Autodesk Fusion 360 part; units mm, degrees
note: some values were not read from the file. Set by a fixed rule: which sketch regions a step uses.
(part 57 of 59)
  spline S63 degree 5 poles (29.6298, 3.3854) (29.6276, 3.3871) (29.6234, 3.3904) (29.6169, 3.3953) (29.6084, 3.4019) (29.5977, 3.41) (29.587, 3.4182) (29.5763, 3.4263) (29.5657, 3.4343) (29.555, 3.4424) (29.5444, 3.4504) (29.5338, 3.4584) (29.5232, 3.4663) (29.5127, 3.4742) (29.5021, 3.4821) (29.4915, 3.4899) (29.481, 3.4978) (29.4705, 3.5055) (29.46, 3.5133) (29.4495, 3.521) (29.4391, 3.5287) (29.4286, 3.5363) (29.4182, 3.544) (29.4078, 3.5515) (29.3974, 3.5591) (29.387, 3.5666) (29.3766, 3.5741) (29.3663, 3.5816) (29.356, 3.589) (29.3457, 3.5964) (29.3354, 3.6037) (29.3251, 3.6111) (29.3148, 3.6184) (29.3046, 3.6256) (29.2944, 3.6329) (29.2842, 3.64) (29.274, 3.6472) (29.2638, 3.6543) (29.2537, 3.6614) (29.2435, 3.6685) (29.2334, 3.6755) (29.2233, 3.6825) (29.2132, 3.6895) (29.2032, 3.6964) (29.1932, 3.7033) (29.1831, 3.7102) (29.1731, 3.717) (29.1632, 3.7238) (29.1532, 3.7306) (29.1433, 3.7374) (29.1334, 3.7441) (29.1235, 3.7507) (29.1136, 3.7574) (29.1037, 3.764) (29.0939, 3.7705) (29.0841, 3.7771) (29.0743, 3.7836) (29.0646, 3.7901) (29.0548, 3.7965) (29.0451, 3.8029) (29.0354, 3.8093) (29.0257, 3.8156) (29.016, 3.8219) (29.0064, 3.8282) (28.9968, 3.8344) (28.9872, 3.8407) (28.9776, 3.8468) (28.9681, 3.853) (28.9586, 3.8591) (28.9491, 3.8652) (28.9396, 3.8712) (28.9302, 3.8772) (28.9207, 3.8832) (28.9113, 3.8891) (28.902, 3.895) (28.8926, 3.9009) (28.8833, 3.9068) (28.874, 3.9126) (28.8647, 3.9183) (28.8555, 3.9241) (28.8462, 3.9298) (28.837, 3.9355) (28.8279, 3.9411) (28.8187, 3.9467) (28.8096, 3.9523) (28.8005, 3.9578) (28.7914, 3.9633) (28.7824, 3.9688) (28.7734, 3.9743) (28.7644, 3.9797) (28.7554, 3.985) (28.7465, 3.9904) (28.7376, 3.9957) (28.7287, 4.001) (28.7199, 4.0062) (28.711, 4.0114) (28.7022, 4.0166) (28.6935, 4.0217) (28.6847, 4.0268) (28.676, 4.0319) (28.6674, 4.037) (28.6587, 4.042) (28.6501, 4.0469) (28.6415, 4.0519) (28.633, 4.0568) (28.6244, 4.0616) (28.616, 4.0665) (28.6075, 4.0713) (28.5991, 4.0761) (28.5907, 4.0808) (28.5823, 4.0855) (28.574, 4.0902) (28.5657, 4.0948) (28.5574, 4.0994) (28.5491, 4.104) (28.5409, 4.1085) (28.5328, 4.113) (28.5246, 4.1175) (28.5165, 4.1219) (28.5085, 4.1263) (28.5004, 4.1307) (28.4924, 4.135) (28.4845, 4.1393) (28.4765, 4.1435) (28.4686, 4.1478) (28.4608, 4.152) (28.4529, 4.1561) (28.4452, 4.1602) (28.4374, 4.1643) (28.4297, 4.1684) (28.422, 4.1724) (28.4144, 4.1764) (28.4068, 4.1804) (28.3992, 4.1843) (28.3917, 4.1882) (28.3842, 4.192) (28.3767, 4.1958) (28.3693, 4.1996) (28.3619, 4.2034) (28.3546, 4.2071) (28.3473, 4.2108) (28.3401, 4.2144) (28.3329, 4.218) (28.3257, 4.2216) (28.3186, 4.2252) (28.3115, 4.2287) (28.3044, 4.2322) (28.2974, 4.2356) (28.2905, 4.239) (28.2835, 4.2424) (28.2767, 4.2457) (28.2698, 4.249) (28.263, 4.2523) (28.2563, 4.2555) (28.2496, 4.2588) (28.2429, 4.2619) (28.2363, 4.2651) (28.2298, 4.2682) (28.2233, 4.2712) (28.2168, 4.2743) (28.2104, 4.2773) (28.204, 4.2802) (28.1977, 4.2831) (28.1914, 4.286) (28.1851, 4.2889) (28.179, 4.2917) (28.1728, 4.2945) (28.1667, 4.2973) (28.1607, 4.3) (28.1547, 4.3027) (28.1488, 4.3053) (28.1429, 4.308) (28.1371, 4.3105) (28.1313, 4.3131) (28.1256, 4.3156) (28.1199, 4.3181) (28.1143, 4.3205) (28.1087, 4.323) (28.1032, 4.3253) (28.0978, 4.3277) (28.0924, 4.33) (28.087, 4.3323) (28.0818, 4.3345) (28.0765, 4.3367) (28.0714, 4.3389) (28.0663, 4.341) (28.0612, 4.3431) (28.0562, 4.3452) (28.0513, 4.3472) (28.0464, 4.3492) (28.0416, 4.3512) (28.0369, 4.3531) (28.0322, 4.355) (28.0276, 4.3568) (28.023, 4.3587) (28.0185, 4.3605) (28.0141, 4.3622) (28.0097, 4.3639) (28.0054, 4.3656) (28.0012, 4.3673) (27.997, 4.3689) (27.9929, 4.3705) (27.9889, 4.372) (27.9849, 4.3735) (27.9811, 4.375) (27.9772, 4.3764) (27.9735, 4.3778) (27.9698, 4.3792) (27.9662, 4.3806) (27.9627, 4.3819) (27.9593, 4.3831) (27.9559, 4.3844) (27.9526, 4.3856) (27.9494, 4.3867) (27.9462, 4.3879) (27.9432, 4.3889) (27.9402, 4.39) (27.9373, 4.391) (27.9345, 4.392) (27.9318, 4.393) (27.9291, 4.3939) (27.9265, 4.3948) (27.9241, 4.3956) (27.9217, 4.3964) (27.9194, 4.3972) (27.9172, 4.398) (27.915, 4.3987) (27.913, 4.3993) (27.9111, 4.4) (27.9092, 4.4006) (27.9075, 4.4012) (27.9058, 4.4017) (27.9043, 4.4022) (27.9028, 4.4027) (27.9015, 4.4031) (27.9002, 4.4035) (27.8991, 4.4038) (27.898, 4.4042) (27.8971, 4.4044) (27.8963, 4.4047) (27.8956, 4.4049) (27.8951, 4.4051) (27.8948, 4.4052) (27.8946, 4.4052) (27.8945, 4.4052) knots -1 -1 -1 -1 -1 -1 -0.99583333 -0.99166667 -0.9875 -0.98333333 -0.97916667 -0.975 -0.97083333 -0.96666667 -0.9625 -0.95833333 -0.95416667 -0.95 -0.94583333 -0.94166667 -0.9375 -0.93333333 -0.92916667 -0.925 -0.92083333 -0.91666667 -0.9125 -0.90833333 -0.90416667 -0.9 -0.89583333 -0.89166667 -0.8875 -0.88333333 -0.87916667 -0.875 -0.87083333 -0.86666667 -0.8625 -0.85833333 -0.85416667 -0.85 -0.84583333 -0.84166667 -0.8375 -0.83333333 -0.82916667 -0.825 -0.82083333 -0.81666667 -0.8125 -0.80833333 -0.80416667 -0.8 -0.79583333 -0.79166667 -0.7875 -0.78333333 -0.77916667 -0.775 -0.77083333 -0.76666667 -0.7625 -0.75833333 -0.75416667 -0.75 -0.74583333 -0.74166667 -0.7375 -0.73333333 -0.72916667 -0.725 -0.72083333 -0.71666667 -0.7125 -0.70833333 -0.70416667 -0.7 -0.69583333 -0.69166667 -0.6875 -0.68333333 -0.67916667 -0.675 -0.67083333 -0.66666667 -0.6625 -0.65833333 -0.65416667 -0.65 -0.64583333 -0.64166667 -0.6375 -0.63333333 -0.62916667 -0.625 -0.62083333 -0.61666667 -0.6125 -0.60833333 -0.60416667 -0.6 -0.59583333 -0.59166667 -0.5875 -0.58333333 -0.57916667 -0.575 -0.57083333 -0.56666667 -0.5625 -0.55833333 -0.55416667 -0.55 -0.54583333 -0.54166667 -0.5375 -0.53333333 -0.52916667 -0.525 -0.52083333 -0.51666667 -0.5125 -0.50833333 -0.50416667 -0.5 -0.49583333 -0.49166667 -0.4875 -0.48333333 -0.47916667 -0.475 -0.47083333 -0.46666667 -0.4625 -0.45833333 -0.45416667 -0.45 -0.44583333 -0.44166667 -0.4375 -0.43333333 -0.42916667 -0.425 -0.42083333 -0.41666667 -0.4125 -0.40833333 -0.40416667 -0.4 -0.39583333 -0.39166667 -0.3875 -0.38333333 -0.37916667 -0.375 -0.37083333 -0.36666667 -0.3625 -0.35833333 -0.35416667 -0.35 -0.34583333 -0.34166667 -0.3375 -0.33333333 -0.32916667 -0.325 -0.32083333 -0.31666667 -0.3125 -0.30833333 -0.30416667 -0.3 -0.29583333 -0.29166667 -0.2875 -0.28333333 -0.27916667 -0.275 -0.27083333 -0.26666667 -0.2625 -0.25833333 -0.25416667 -0.25 -0.24583333 -0.24166667 -0.2375 -0.23333333 -0.22916667 -0.225 -0.22083333 -0.21666667 -0.2125 -0.20833333 -0.20416667 -0.2 -0.19583333 -0.19166667 -0.1875 -0.18333333 -0.17916667 -0.175 -0.17083333 -0.16666667 -0.1625 -0.15833333 -0.15416667 -0.15 -0.14583333 -0.14166667 -0.1375 -0.13333333 -0.12916667 -0.125 -0.12083333 -0.11666667 -0.1125 -0.10833333 -0.10416667 -0.1 -0.09583333 -0.09166667 -0.0875 -0.08333333 -0.07916667 -0.075 -0.07083333 -0.06666667 -0.0625 -0.05833333 -0.05416667 -0.05 -0.04583333 -0.04166667 -0.0375 -0.03333333 -0.02916667 -0.025 -0.02083333 -0.01666667 -0.0125 -0.00833333 -0.00416667 0 0 0 0 0 0
  line L127 (27.8945, 4.4052) -> (27.8937, 4.4055)
  line L128 (27.8937, 4.4055) -> (27.6109, 4.4875)
  arc A64 (27.6109, 4.4875) -> (27.918, 5.6335) centre (0, 12.5) ccw
  line L129 (27.918, 5.6335) -> (28.2039, 5.5632)
  line L130 (28.2039, 5.5632) -> (28.2047, 5.563)
  spline S64 degree 5 poles (28.2047, 5.563) (28.2048, 5.563) (28.205, 5.563) (28.2053, 5.5629) (28.2058, 5.5628) (28.2065, 5.5626) (28.2074, 5.5624) (28.2083, 5.5622) (28.2094, 5.5619) (28.2106, 5.5617) (28.2118, 5.5614) (28.2132, 5.5611) (28.2147, 5.5608) (28.2163, 5.5604) (28.218, 5.5601) (28.2198, 5.5597) (28.2217, 5.5593) (28.2237, 5.5589) (28.2258, 5.5584) (28.228, 5.558) (28.2303, 5.5575) (28.2327, 5.5571) (28.2351, 5.5566) (28.2377, 5.5561) (28.2404, 5.5555) (28.2431, 5.555) (28.246, 5.5545) (28.2489, 5.5539) (28.2519, 5.5534) (28.255, 5.5528) (28.2582, 5.5522) (28.2615, 5.5516) (28.2649, 5.551) (28.2683, 5.5504) (28.2719, 5.5498) (28.2755, 5.5492) (28.2792, 5.5485) (28.283, 5.5479) (28.2868, 5.5472) (28.2908, 5.5466) (28.2948, 5.5459) (28.2989, 5.5453) (28.3031, 5.5446) (28.3074, 5.5439) (28.3117, 5.5432) (28.3161, 5.5426) (28.3206, 5.5419) (28.3252, 5.5412) (28.3298, 5.5405) (28.3345, 5.5398) (28.3393, 5.5391) (28.3442, 5.5384) (28.3491, 5.5377) (28.3541, 5.537) (28.3592, 5.5363) (28.3643, 5.5356) (28.3695, 5.5349) (28.3748, 5.5342) (28.3802, 5.5335) (28.3856, 5.5328) (28.3911, 5.5321) (28.3966, 5.5314) (28.4023, 5.5307) (28.408, 5.53) (28.4137, 5.5293) (28.4196, 5.5286) (28.4255, 5.5279) (28.4314, 5.5272) (28.4374, 5.5265) (28.4435, 5.5258) (28.4497, 5.5251) (28.4559, 5.5244) (28.4622, 5.5237) (28.4685, 5.5231) (28.4749, 5.5224) (28.4814, 5.5217) (28.4879, 5.5211) (28.4945, 5.5204) (28.5011, 5.5197) (28.5078, 5.5191) (28.5146, 5.5184) (28.5214, 5.5178) (28.5283, 5.5172) (28.5353, 5.5165) (28.5423, 5.5159) (28.5493, 5.5153) (28.5564, 5.5147) (28.5636, 5.5141) (28.5709, 5.5135) (28.5781, 5.5129) (28.5855, 5.5123) (28.5929, 5.5118) (28.6004, 5.5112) (28.6079, 5.5106) (28.6154, 5.5101) (28.6231, 5.5095) (28.6307, 5.509) (28.6385, 5.5085) (28.6463, 5.5079) (28.6541, 5.5074) (28.662, 5.5069) (28.67, 5.5064) (28.678, 5.506) (28.686, 5.5055) (28.6941, 5.505) (28.7023, 5.5046) (28.7105, 5.5041) (28.7187, 5.5037) (28.727, 5.5032) (28.7354, 5.5028) (28.7438, 5.5024) (28.7523, 5.502) (28.7608, 5.5016) (28.7694, 5.5013) (28.778, 5.5009) (28.7866, 5.5005) (28.7953, 5.5002) (28.8041, 5.4999) (28.8129, 5.4995) (28.8218, 5.4992) (28.8307, 5.4989) (28.8396, 5.4986) (28.8486, 5.4984) (28.8577, 5.4981) (28.8668, 5.4979) (28.8759, 5.4976) (28.8851, 5.4974) (28.8943, 5.4972) (28.9036, 5.497) (28.9129, 5.4968) (28.9223, 5.4966) (28.9317, 5.4964) (28.9412, 5.4963) (28.9507, 5.4962) (28.9602, 5.496) (28.9698, 5.4959) (28.9795, 5.4958) (28.9892, 5.4957) (28.9989, 5.4957) (29.0087, 5.4956) (29.0185, 5.4956) (29.0284, 5.4955) (29.0383, 5.4955) (29.0482, 5.4955) (29.0582, 5.4955) (29.0682, 5.4956) (29.0783, 5.4956) (29.0884, 5.4957) (29.0986, 5.4957) (29.1088, 5.4958) (29.119, 5.4959) (29.1293, 5.496) (29.1396, 5.4962) (29.15, 5.4963) (29.1604, 5.4965) (29.1708, 5.4966) (29.1813, 5.4968) (29.1919, 5.497) (29.2024, 5.4972) (29.213, 5.4975) (29.2237, 5.4977) (29.2344, 5.498) (29.2451, 5.4983) (29.2559, 5.4986) (29.2667, 5.4989) (29.2775, 5.4992) (29.2884, 5.4996) (29.2993, 5.4999) (29.3103, 5.5003) (29.3213, 5.5007) (29.3323, 5.5011) (29.3434, 5.5016) (29.3545, 5.502) (29.3657, 5.5025) (29.3768, 5.503) (29.3881, 5.5035) (29.3993, 5.504) (29.4106, 5.5045) (29.422, 5.505) (29.4333, 5.5056) (29.4447, 5.5062) (29.4562, 5.5068) (29.4677, 5.5074) (29.4792, 5.508) (29.4907, 5.5087) (29.5023, 5.5094) (29.514, 5.51) (29.5256, 5.5108) (29.5373, 5.5115) (29.549, 5.5122) (29.5608, 5.513) (29.5726, 5.5137) (29.5844, 5.5145) (29.5963, 5.5154) (29.6082, 5.5162) (29.6201, 5.517) (29.6321, 5.5179) (29.6441, 5.5188) (29.6562, 5.5197) (29.6682, 5.5206) (29.6803, 5.5216) (29.6925, 5.5225) (29.7047, 5.5235) (29.7169, 5.5245) (29.7291, 5.5255) (29.7414, 5.5265) (29.7537, 5.5276) (29.766, 5.5287) (29.7784, 5.5298) (29.7908, 5.5309) (29.8032, 5.532) (29.8157, 5.5331) (29.8282, 5.5343) (29.8407, 5.5355) (29.8533, 5.5367) (29.8659, 5.5379) (29.8785, 5.5392) (29.8912, 5.5404) (29.9039, 5.5417) (29.9166, 5.543) (29.9293, 5.5444) (29.9421, 5.5457) (29.9549, 5.5471) (29.9678, 5.5484) (29.9806, 5.5499) (29.9935, 5.5513) (30.0065, 5.5527) (30.0194, 5.5542) (30.0324, 5.5557) (30.0455, 5.5572) (30.0585, 5.5587) (30.0716, 5.5602) (30.0847, 5.5618) (30.0979, 5.5634) (30.111, 5.565) (30.1242, 5.5666) (30.1375, 5.5683) (30.1507, 5.5699) (30.164, 5.5716) (30.1773, 5.5733) (30.1907, 5.575) (30.2014, 5.5764) (30.2094, 5.5775) (30.2148, 5.5782) (30.2174, 5.5786) knots 0 0 0 0 0 0 0.00416667 0.00833333 0.0125 0.01666667 0.02083333 0.025 0.02916667 0.03333333 0.0375 0.04166667 0.04583333 0.05 0.05416667 0.05833333 0.0625 0.06666667 0.07083333 0.075 0.07916667 0.08333333 0.0875 0.09166667 0.09583333 0.1 0.10416667 0.10833333 0.1125 0.11666667 0.12083333 0.125 0.12916667 0.13333333 0.1375 0.14166667 0.14583333 0.15 0.15416667 0.15833333 0.1625 0.16666667 0.17083333 0.175 0.17916667 0.18333333 0.1875 0.19166667 0.19583333 0.2 0.20416667 0.20833333 0.2125 0.21666667 0.22083333 0.225 0.22916667 0.23333333 0.2375 0.24166667 0.24583333 0.25 0.25416667 0.25833333 0.2625 0.26666667 0.27083333 0.275 0.27916667 0.28333333 0.2875 0.29166667 0.29583333 0.3 0.30416667 0.30833333 0.3125 0.31666667 0.32083333 0.325 0.32916667 0.33333333 0.3375 0.34166667 0.34583333 0.35 0.35416667 0.35833333 0.3625 0.36666667 0.37083333 0.375 0.37916667 0.38333333 0.3875 0.39166667 0.39583333 0.4 0.40416667 0.40833333 0.4125 0.41666667 0.42083333 0.425 0.42916667 0.43333333 0.4375 0.44166667 0.44583333 0.45 0.45416667 0.45833333 0.4625 0.46666667 0.47083333 0.475 0.47916667 0.48333333 0.4875 0.49166667 0.49583333 0.5 0.50416667 0.50833333 0.5125 0.51666667 0.52083333 0.525 0.52916667 0.53333333 0.5375 0.54166667 0.54583333 0.55 0.55416667 0.55833333 0.5625 0.56666667 0.57083333 0.575 0.57916667 0.58333333 0.5875 0.59166667 0.59583333 0.6 0.60416667 0.60833333 0.6125 0.61666667 0.62083333 0.625 0.62916667 0.63333333 0.6375 0.64166667 0.64583333 0.65 0.65416667 0.65833333 0.6625 0.66666667 0.67083333 0.675 0.67916667 0.68333333 0.6875 0.69166667 0.69583333 0.7 0.70416667 0.70833333 0.7125 0.71666667 0.72083333 0.725 0.72916667 0.73333333 0.7375 0.74166667 0.74583333 0.75 0.75416667 0.75833333 0.7625 0.76666667 0.77083333 0.775 0.77916667 0.78333333 0.7875 0.79166667 0.79583333 0.8 0.80416667 0.80833333 0.8125 0.81666667 0.82083333 0.825 0.82916667 0.83333333 0.8375 0.84166667 0.84583333 0.85 0.85416667 0.85833333 0.8625 0.86666667 0.87083333 0.875 0.87916667 0.88333333 0.8875 0.89166667 0.89583333 0.9 0.90416667 0.90833333 0.9125 0.91666667 0.92083333 0.925 0.92916667 0.93333333 0.9375 0.94166667 0.94583333 0.95 0.95416667 0.95833333 0.9625 0.96666667 0.97083333 0.975 0.97916667 0.98333333 0.9875 0.99166667 0.99583333 1 1 1 1 1 1
  arc A65 (30.2174, 5.5786) -> (30.4202, 6.5325) centre (0, 12.5) ccw
  spline S65 degree 5 poles (30.4202, 6.5325) (30.4179, 6.5339) (30.4133, 6.5367) (30.4064, 6.541) (30.3972, 6.5466) (30.3857, 6.5536) (30.3742, 6.5606) (30.3628, 6.5675) (30.3513, 6.5745) (30.3399, 6.5813) (30.3285, 6.5882) (30.3171, 6.595) (30.3058, 6.6018) (30.2944, 6.6086) (30.2831, 6.6153) (30.2718, 6.622) (30.2605, 6.6287) (30.2492, 6.6353) (30.238, 6.6419) (30.2268, 6.6485) (30.2156, 6.6551) (30.2044, 6.6616) (30.1932, 6.6681) (30.1821, 6.6745) (30.1709, 6.6809) (30.1598, 6.6873) (30.1487, 6.6937) (30.1377, 6.7) (30.1266, 6.7063) (30.1156, 6.7126) (30.1046, 6.7189) (30.0936, 6.7251) (30.0826, 6.7312) (30.0717, 6.7374) (30.0608, 6.7435) (30.0499, 6.7496) (30.039, 6.7557) (30.0281, 6.7617) (30.0173, 6.7677) (30.0065, 6.7737) (29.9957, 6.7796) (29.9849, 6.7855) (29.9742, 6.7914) (29.9634, 6.7972) (29.9527, 6.803) (29.9421, 6.8088) (29.9314, 6.8146) (29.9208, 6.8203) (29.9102, 6.826) (29.8996, 6.8317) (29.889, 6.8373) (29.8785, 6.8429) (29.868, 6.8485) (29.8575, 6.854) (29.847, 6.8595) (29.8366, 6.865) (29.8262, 6.8704) (29.8158, 6.8758) (29.8054, 6.8812) (29.7951, 6.8866) (29.7847, 6.8919) (29.7745, 6.8972) (29.7642, 6.9025) (29.754, 6.9077) (29.7437, 6.9129) (29.7336, 6.9181) (29.7234, 6.9232) (29.7133, 6.9283) (29.7032, 6.9334) (29.6931, 6.9385) (29.683, 6.9435) (29.673, 6.9485) (29.663, 6.9534) (29.653, 6.9584) (29.6431, 6.9633) (29.6332, 6.9681) (29.6233, 6.973) (29.6134, 6.9778) (29.6036, 6.9825) (29.5938, 6.9873) (29.584, 6.992) (29.5743, 6.9967) (29.5646, 7.0013) (29.5549, 7.006) (29.5452, 7.0105) (29.5356, 7.0151) (29.526, 7.0196) (29.5165, 7.0241) (29.5069, 7.0286) (29.4974, 7.033) (29.4879, 7.0375) (29.4785, 7.0418) (29.4691, 7.0462) (29.4597, 7.0505) (29.4504, 7.0548) (29.441, 7.059) (29.4318, 7.0633) (29.4225, 7.0675) (29.4133, 7.0716) (29.4041, 7.0758) (29.395, 7.0799) (29.3858, 7.0839) (29.3767, 7.088) (29.3677, 7.092) (29.3587, 7.096) (29.3497, 7.0999) (29.3407, 7.1039) (29.3318, 7.1078) (29.3229, 7.1116) (29.3141, 7.1154) (29.3053, 7.1193) (29.2965, 7.123) (29.2878, 7.1268) (29.279, 7.1305) (29.2704, 7.1342) (29.2617, 7.1378) (29.2531, 7.1414) (29.2446, 7.145) (29.2361, 7.1486) (29.2276, 7.1521) (29.2191, 7.1556) (29.2107, 7.1591) (29.2023, 7.1625) (29.194, 7.1659) (29.1857, 7.1693) (29.1775, 7.1727) (29.1692, 7.176) (29.1611, 7.1793) (29.1529, 7.1825) (29.1448, 7.1857) (29.1368, 7.1889) (29.1288, 7.1921) (29.1208, 7.1953) (29.1129, 7.1984) (29.105, 7.2014) (29.0971, 7.2045) (29.0893, 7.2075) (29.0815, 7.2105) (29.0738, 7.2135) (29.0661, 7.2164) (29.0585, 7.2193) (29.0509, 7.2222) (29.0433, 7.225) (29.0358, 7.2278) (29.0284, 7.2306) (29.021, 7.2334) (29.0136, 7.2361) (29.0063, 7.2388) (28.999, 7.2414) (28.9918, 7.2441) (28.9846, 7.2467) (28.9774, 7.2492) (28.9703, 7.2518) (28.9633, 7.2543) (28.9563, 7.2568) (28.9493, 7.2592) (28.9424, 7.2617) (28.9356, 7.2641) (28.9288, 7.2664) (28.922, 7.2688) (28.9153, 7.2711) (28.9087, 7.2734) (28.9021, 7.2756) (28.8955, 7.2778) (28.889, 7.28) (28.8826, 7.2822) (28.8762, 7.2843) (28.8699, 7.2864) (28.8636, 7.2885) (28.8573, 7.2906) (28.8512, 7.2926) (28.8451, 7.2946) (28.839, 7.2965) (28.833, 7.2985) (28.827, 7.3004) (28.8211, 7.3022) (28.8153, 7.3041) (28.8095, 7.3059) (28.8038, 7.3077) (28.7981, 7.3095) (28.7925, 7.3112) (28.7869, 7.3129) (28.7815, 7.3146) (28.776, 7.3162) (28.7707, 7.3178) (28.7654, 7.3194) (28.7601, 7.321) (28.7549, 7.3225) (28.7498, 7.324) (28.7448, 7.3255) (28.7398, 7.327) (28.7349, 7.3284) (28.73, 7.3298) (28.7252, 7.3311) (28.7205, 7.3325) (28.7158, 7.3338) (28.7112, 7.3351) (28.7067, 7.3363) (28.7023, 7.3375) (28.6979, 7.3387) (28.6936, 7.3399) (28.6893, 7.3411) (28.6852, 7.3422) (28.6811, 7.3433) (28.6771, 7.3443) (28.6731, 7.3454) (28.6693, 7.3464) (28.6655, 7.3473) (28.6617, 7.3483) (28.6581, 7.3492) (28.6545, 7.3501) (28.6511, 7.351) (28.6477, 7.3519) (28.6443, 7.3527) (28.6411, 7.3535) (28.6379, 7.3542) (28.6349, 7.355) (28.6319, 7.3557) (28.629, 7.3564) (28.6262, 7.357) (28.6234, 7.3577) (28.6208, 7.3583) (28.6182, 7.3589) (28.6158, 7.3594) (28.6134, 7.36) (28.6111, 7.3605) (28.6089, 7.361) (28.6069, 7.3614) (28.6049, 7.3619) (28.603, 7.3623) (28.6012, 7.3626) (28.5995, 7.363) (28.5979, 7.3633) (28.5964, 7.3637) (28.595, 7.3639) (28.5937, 7.3642) (28.5925, 7.3644) (28.5915, 7.3646) (28.5905, 7.3648) (28.5896, 7.365) (28.5889, 7.3651) (28.5884, 7.3652) (28.5881, 7.3653) (28.5879, 7.3653) (28.5878, 7.3654) knots -1 -1 -1 -1 -1 -1 -0.99583333 -0.99166667 -0.9875 -0.98333333 -0.97916667 -0.975 -0.97083333 -0.96666667 -0.9625 -0.95833333 -0.95416667 -0.95 -0.94583333 -0.94166667 -0.9375 -0.93333333 -0.92916667 -0.925 -0.92083333 -0.91666667 -0.9125 -0.90833333 -0.90416667 -0.9 -0.89583333 -0.89166667 -0.8875 -0.88333333 -0.87916667 -0.875 -0.87083333 -0.86666667 -0.8625 -0.85833333 -0.85416667 -0.85 -0.84583333 -0.84166667 -0.8375 -0.83333333 -0.82916667 -0.825 -0.82083333 -0.81666667 -0.8125 -0.80833333 -0.80416667 -0.8 -0.79583333 -0.79166667 -0.7875 -0.78333333 -0.77916667 -0.775 -0.77083333 -0.76666667 -0.7625 -0.75833333 -0.75416667 -0.75 -0.74583333 -0.74166667 -0.7375 -0.73333333 -0.72916667 -0.725 -0.72083333 -0.71666667 -0.7125 -0.70833333 -0.70416667 -0.7 -0.69583333 -0.69166667 -0.6875 -0.68333333 -0.67916667 -0.675 -0.67083333 -0.66666667 -0.6625 -0.65833333 -0.65416667 -0.65 -0.64583333 -0.64166667 -0.6375 -0.63333333 -0.62916667 -0.625 -0.62083333 -0.61666667 -0.6125 -0.60833333 -0.60416667 -0.6 -0.59583333 -0.59166667 -0.5875 -0.58333333 -0.57916667 -0.575 -0.57083333 -0.56666667 -0.5625 -0.55833333 -0.55416667 -0.55 -0.54583333 -0.54166667 -0.5375 -0.53333333 -0.52916667 -0.525 -0.52083333 -0.51666667 -0.5125 -0.50833333 -0.50416667 -0.5 -0.49583333 -0.49166667 -0.4875 -0.48333333 -0.47916667 -0.475 -0.47083333 -0.46666667 -0.4625 -0.45833333 -0.45416667 -0.45 -0.44583333 -0.44166667 -0.4375 -0.43333333 -0.42916667 -0.425 -0.42083333 -0.41666667 -0.4125 -0.40833333 -0.40416667 -0.4 -0.39583333 -0.39166667 -0.3875 -0.38333333 -0.37916667 -0.375 -0.37083333 -0.36666667 -0.3625 -0.35833333 -0.35416667 -0.35 -0.34583333 -0.34166667 -0.3375 -0.33333333 -0.32916667 -0.325 -0.32083333 -0.31666667 -0.3125 -0.30833333 -0.30416667 -0.3 -0.29583333 -0.29166667 -0.2875 -0.28333333 -0.27916667 -0.275 -0.27083333 -0.26666667 -0.2625 -0.25833333 -0.25416667 -0.25 -0.24583333 -0.24166667 -0.2375 -0.23333333 -0.22916667 -0.225 -0.22083333 -0.21666667 -0.2125 -0.20833333 -0.20416667 -0.2 -0.19583333 -0.19166667 -0.1875 -0.18333333 -0.17916667 -0.175 -0.17083333 -0.16666667 -0.1625 -0.15833333 -0.15416667 -0.15 -0.14583333 -0.14166667 -0.1375 -0.13333333 -0.12916667 -0.125 -0.12083333 -0.11666667 -0.1125 -0.10833333 -0.10416667 -0.1 -0.09583333 -0.09166667 -0.0875 -0.08333333 -0.07916667 -0.075 -0.07083333 -0.06666667 -0.0625 -0.05833333 -0.05416667 -0.05 -0.04583333 -0.04166667 -0.0375 -0.03333333 -0.02916667 -0.025 -0.02083333 -0.01666667 -0.0125 -0.00833333 -0.00416667 0 0 0 0 0 0
  line L131 (28.5878, 7.3654) -> (28.587, 7.3655)
  line L132 (28.587, 7.3655) -> (28.2972, 7.4176)
  arc A66 (28.2972, 7.4176) -> (28.4828, 8.5894) centre (0, 12.5) ccw
  line L133 (28.4828, 8.5894) -> (28.7745, 8.5493)
  line L134 (28.7745, 8.5493) -> (28.7753, 8.5492)
  spline S66 degree 5 poles (28.7753, 8.5492) (28.7754, 8.5492) (28.7756, 8.5492) (28.7759, 8.5491) (28.7764, 8.5491) (28.7772, 8.549) (28.778, 8.5489) (28.779, 8.5488) (28.7801, 8.5486) (28.7813, 8.5485) (28.7826, 8.5483) (28.784, 8.5482) (28.7855, 8.548) (28.7871, 8.5478) (28.7889, 8.5477) (28.7907, 8.5475) (28.7926, 8.5473) (28.7946, 8.5471) (28.7968, 8.5469) (28.799, 8.5466) (28.8013, 8.5464) (28.8037, 8.5462) (28.8063, 8.546) (28.8089, 8.5457) (28.8116, 8.5455) (28.8144, 8.5453) (28.8172, 8.545) (28.8202, 8.5448) (28.8233, 8.5445) (28.8264, 8.5443) (28.8297, 8.5441) (28.833, 8.5438) (28.8364, 8.5436) (28.8399, 8.5433) (28.8435, 8.5431) (28.8472, 8.5428) (28.8509, 8.5426) (28.8547, 8.5423) (28.8586, 8.5421) (28.8626, 8.5419) (28.8667, 8.5416) (28.8709, 8.5414) (28.8751, 8.5412) (28.8794, 8.541) (28.8838, 8.5407) (28.8882, 8.5405) (28.8928, 8.5403) (28.8974, 8.5401) (28.9021, 8.5399) (28.9068, 8.5397) (28.9117, 8.5395) (28.9166, 8.5393) (28.9215, 8.5391) (28.9266, 8.539) (28.9317, 8.5388) (28.9369, 8.5386) (28.9422, 8.5385) (28.9475, 8.5383) (28.9529, 8.5382) (28.9584, 8.538) (28.9639, 8.5379) (28.9695, 8.5378) (28.9752, 8.5377) (28.9809, 8.5376) (28.9867, 8.5375) (28.9926, 8.5374) (28.9985, 8.5373) (29.0045, 8.5373) (29.0106, 8.5372) (29.0167, 8.5371) (29.0229, 8.5371) (29.0291, 8.5371) (29.0355, 8.5371) (29.0418, 8.537) (29.0483, 8.537) (29.0548, 8.5371) (29.0613, 8.5371) (29.068, 8.5371) (29.0746, 8.5372) (29.0814, 8.5372) (29.0882, 8.5373) (29.095, 8.5374) (29.1019, 8.5374) (29.1089, 8.5375) (29.1159, 8.5377) (29.123, 8.5378) (29.1302, 8.5379) (29.1374, 8.5381) (29.1446, 8.5382) (29.1519, 8.5384) (29.1593, 8.5386) (29.1667, 8.5388) (29.1742, 8.539) (29.1817, 8.5393) (29.1893, 8.5395) (29.197, 8.5397) (29.2047, 8.54) (29.2124, 8.5403) (29.2202, 8.5406) (29.2281, 8.5409) (29.236, 8.5412) (29.2439, 8.5416) (29.2519, 8.5419) (29.26, 8.5423) (29.2681, 8.5427) (29.2763, 8.5431) (29.2845, 8.5435) (29.2927, 8.5439) (29.301, 8.5444) (29.3094, 8.5448) (29.3178, 8.5453) (29.3263, 8.5458) (29.3348, 8.5463) (29.3433, 8.5468) (29.3519, 8.5474) (29.3606, 8.5479) (29.3693, 8.5485) (29.378, 8.5491) (29.3868, 8.5497) (29.3957, 8.5503) (29.4045, 8.5509) (29.4135, 8.5516) (29.4225, 8.5522) (29.4315, 8.5529) (29.4406, 8.5536) (29.4497, 8.5543) (29.4588, 8.5551) (29.468, 8.5558) (29.4773, 8.5566) (29.4866, 8.5574) (29.4959, 8.5582) (29.5053, 8.559) (29.5147, 8.5598) (29.5242, 8.5607) (29.5337, 8.5616) (29.5433, 8.5625) (29.5529, 8.5634) (29.5625, 8.5643) (29.5722, 8.5652) (29.5819, 8.5662) (29.5917, 8.5672) (29.6015, 8.5682) (29.6113, 8.5692) (29.6212, 8.5703) (29.6312, 8.5713) (29.6411, 8.5724) (29.6512, 8.5735) (29.6612, 8.5746) (29.6713, 8.5757) (29.6814, 8.5769) (29.6916, 8.578) (29.7018, 8.5792) (29.7121, 8.5804) (29.7224, 8.5817) (29.7327, 8.5829) (29.7431, 8.5842) (29.7535, 8.5855) (29.764, 8.5868) (29.7744, 8.5881) (29.785, 8.5894) (29.7955, 8.5908) (29.8061, 8.5922) (29.8168, 8.5936) (29.8274, 8.595) (29.8382, 8.5965) (29.8489, 8.5979) (29.8597, 8.5994) (29.8705, 8.6009) (29.8814, 8.6024) (29.8923, 8.604) (29.9032, 8.6055) (29.9142, 8.6071) (29.9252, 8.6087) (29.9362, 8.6104) (29.9473, 8.612) (29.9584, 8.6137) (29.9696, 8.6154) (29.9807, 8.6171) (29.992, 8.6188) (30.0032, 8.6205) (30.0145, 8.6223) (30.0258, 8.6241) (30.0372, 8.6259) (30.0486, 8.6278) (30.06, 8.6296) (30.0714, 8.6315) (30.0829, 8.6334) (30.0944, 8.6353) (30.106, 8.6372) (30.1176, 8.6392) (30.1292, 8.6412) (30.1409, 8.6432) (30.1525, 8.6452) (30.1643, 8.6473) (30.176, 8.6493) (30.1878, 8.6514) (30.1996, 8.6536) (30.2115, 8.6557) (30.2233, 8.6578) (30.2353, 8.66) (30.2472, 8.6622) (30.2592, 8.6644) (30.2712, 8.6667) (30.2832, 8.669) (30.2953, 8.6712) (30.3074, 8.6736) (30.3195, 8.6759) (30.3317, 8.6783) (30.3439, 8.6806) (30.3561, 8.683) (30.3683, 8.6855) (30.3806, 8.6879) (30.3929, 8.6904) (30.4053, 8.6929) (30.4176, 8.6954) (30.43, 8.6979) (30.4424, 8.7005) (30.4549, 8.703) (30.4674, 8.7057) (30.4799, 8.7083) (30.4924, 8.7109) (30.505, 8.7136) (30.5176, 8.7163) (30.5302, 8.719) (30.5429, 8.7218) (30.5556, 8.7245) (30.5683, 8.7273) (30.581, 8.7301) (30.5938, 8.733) (30.6066, 8.7358) (30.6194, 8.7387) (30.6323, 8.7416) (30.6451, 8.7445) (30.658, 8.7475) (30.671, 8.7504) (30.6839, 8.7534) (30.6969, 8.7565) (30.7099, 8.7595) (30.723, 8.7626) (30.736, 8.7657) (30.7491, 8.7688) (30.7596, 8.7713) (30.7675, 8.7732) (30.7728, 8.7744) (30.7754, 8.7751) knots 0 0 0 0 0 0 0.00416667 0.00833333 0.0125 0.01666667 0.02083333 0.025 0.02916667 0.03333333 0.0375 0.04166667 0.04583333 0.05 0.05416667 0.05833333 0.0625 0.06666667 0.07083333 0.075 0.07916667 0.08333333 0.0875 0.09166667 0.09583333 0.1 0.10416667 0.10833333 0.1125 0.11666667 0.12083333 0.125 0.12916667 0.13333333 0.1375 0.14166667 0.14583333 0.15 0.15416667 0.15833333 0.1625 0.16666667 0.17083333 0.175 0.17916667 0.18333333 0.1875 0.19166667 0.19583333 0.2 0.20416667 0.20833333 0.2125 0.21666667 0.22083333 0.225 0.22916667 0.23333333 0.2375 0.24166667 0.24583333 0.25 0.25416667 0.25833333 0.2625 0.26666667 0.27083333 0.275 0.27916667 0.28333333 0.2875 0.29166667 0.29583333 0.3 0.30416667 0.30833333 0.3125 0.31666667 0.32083333 0.325 0.32916667 0.33333333 0.3375 0.34166667 0.34583333 0.35 0.35416667 0.35833333 0.3625 0.36666667 0.37083333 0.375 0.37916667 0.38333333 0.3875 0.39166667 0.39583333 0.4 0.40416667 0.40833333 0.4125 0.41666667 0.42083333 0.425 0.42916667 0.43333333 0.4375 0.44166667 0.44583333 0.45 0.45416667 0.45833333 0.4625 0.46666667 0.47083333 0.475 0.47916667 0.48333333 0.4875 0.49166667 0.49583333 0.5 0.50416667 0.50833333 0.5125 0.51666667 0.52083333 0.525 0.52916667 0.53333333 0.5375 0.54166667 0.54583333 0.55 0.55416667 0.55833333 0.5625 0.56666667 0.57083333 0.575 0.57916667 0.58333333 0.5875 0.59166667 0.59583333 0.6 0.60416667 0.60833333 0.6125 0.61666667 0.62083333 0.625 0.62916667 0.63333333 0.6375 0.64166667 0.64583333 0.65 0.65416667 0.65833333 0.6625 0.66666667 0.67083333 0.675 0.67916667 0.68333333 0.6875 0.69166667 0.69583333 0.7 0.70416667 0.70833333 0.7125 0.71666667 0.72083333 0.725 0.72916667 0.73333333 0.7375 0.74166667 0.74583333 0.75 0.75416667 0.75833333 0.7625 0.76666667 0.77083333 0.775 0.77916667 0.78333333 0.7875 0.79166667 0.79583333 0.8 0.80416667 0.80833333 0.8125 0.81666667 0.82083333 0.825 0.82916667 0.83333333 0.8375 0.84166667 0.84583333 0.85 0.85416667 0.85833333 0.8625 0.86666667 0.87083333 0.875 0.87916667 0.88333333 0.8875 0.89166667 0.89583333 0.9 0.90416667 0.90833333 0.9125 0.91666667 0.92083333 0.925 0.92916667 0.93333333 0.9375 0.94166667 0.94583333 0.95 0.95416667 0.95833333 0.9625 0.96666667 0.97083333 0.975 0.97916667 0.98333333 0.9875 0.99166667 0.99583333 1 1 1 1 1 1
  arc A67 (30.7754, 8.7751) -> (30.8773, 9.745) centre (0, 12.5) ccw
  spline S67 degree 5 poles (30.8773, 9.745) (30.8749, 9.7461) (30.87, 9.7485) (30.8627, 9.752) (30.853, 9.7566) (30.8408, 9.7624) (30.8287, 9.7681) (30.8165, 9.7738) (30.8044, 9.7795) (30.7924, 9.7851) (30.7803, 9.7908) (30.7683, 9.7964) (30.7563, 9.8019) (30.7443, 9.8075) (30.7323, 9.813) (30.7204, 9.8185) (30.7085, 9.8239) (30.6966, 9.8293) (30.6847, 9.8347) (30.6728, 9.8401) (30.661, 9.8455) (30.6492, 9.8508) (30.6374, 9.8561) (30.6256, 9.8613) (30.6139, 9.8665) (30.6022, 9.8717) (30.5905, 9.8769) (30.5788, 9.8821) (30.5672, 9.8872) (30.5555, 9.8923) (30.5439, 9.8973) (30.5324, 9.9023) (30.5208, 9.9073) (30.5093, 9.9123) (30.4978, 9.9173) (30.4863, 9.9222) (30.4749, 9.9271) (30.4634, 9.9319) (30.452, 9.9368) (30.4407, 9.9416) (30.4293, 9.9463) (30.418, 9.9511) (30.4067, 9.9558) (30.3954, 9.9605) (30.3841, 9.9652) (30.3729, 9.9698) (30.3617, 9.9744) (30.3506, 9.979) (30.3394, 9.9835) (30.3283, 9.9881) (30.3172, 9.9926) (30.3061, 9.997) (30.2951, 10.0015) (30.2841, 10.0059) (30.2731, 10.0103) (30.2621, 10.0146) (30.2512, 10.019) (30.2403, 10.0233) (30.2294, 10.0275) (30.2186, 10.0318) (30.2078, 10.036) (30.197, 10.0402) (30.1862, 10.0443) (30.1755, 10.0485) (30.1648, 10.0526) (30.1541, 10.0567) (30.1435, 10.0607) (30.1329, 10.0647) (30.1223, 10.0687) (30.1118, 10.0727) (30.1012, 10.0766) (30.0907, 10.0806) (30.0803, 10.0844) (30.0699, 10.0883) (30.0595, 10.0921) (30.0491, 10.0959) (30.0388, 10.0997) (30.0284, 10.1035) (30.0182, 10.1072) (30.0079, 10.1109) (29.9977, 10.1145) (29.9875, 10.1182) (29.9774, 10.1218) (29.9673, 10.1254) (29.9572, 10.1289) (29.9471, 10.1325) (29.9371, 10.136) (29.9271, 10.1394) (29.9172, 10.1429) (29.9073, 10.1463) (29.8974, 10.1497) (29.8875, 10.1531) (29.8777, 10.1564) (29.868, 10.1597) (29.8582, 10.163) (29.8485, 10.1663) (29.8388, 10.1695) (29.8292, 10.1727) (29.8196, 10.1759) (29.81, 10.179) (29.8005, 10.1822) (29.791, 10.1853) (29.7815, 10.1883) (29.7721, 10.1914) (29.7627, 10.1944) (29.7534, 10.1974) (29.7441, 10.2004) (29.7348, 10.2033) (29.7255, 10.2062) (29.7163, 10.2091) (29.7072, 10.212) (29.6981, 10.2148) (29.689, 10.2176) (29.6799, 10.2204) (29.6709, 10.2231) (29.6619, 10.2259) (29.653, 10.2286) (29.6441, 10.2312) (29.6353, 10.2339) (29.6265, 10.2365) (29.6177, 10.2391) (29.609, 10.2417) (29.6003, 10.2442) (29.5917, 10.2467) (29.583, 10.2492) (29.5745, 10.2517) (29.566, 10.2542) (29.5575, 10.2566) (29.5491, 10.259) (29.5407, 10.2613) (29.5323, 10.2637) (29.524, 10.266) (29.5158, 10.2683) (29.5075, 10.2705) (29.4994, 10.2728) (29.4912, 10.275) (29.4832, 10.2772) (29.4751, 10.2793) (29.4671, 10.2815) (29.4592, 10.2836) (29.4513, 10.2857) (29.4434, 10.2877) (29.4356, 10.2898) (29.4279, 10.2918) (29.4202, 10.2938) (29.4125, 10.2957) (29.4049, 10.2977) (29.3973, 10.2996) (29.3898, 10.3015) (29.3823, 10.3033) (29.3749, 10.3052) (29.3675, 10.307) (29.3602, 10.3088) (29.3529, 10.3105) (29.3457, 10.3123) (29.3386, 10.314) (29.3314, 10.3157) (29.3244, 10.3173) (29.3174, 10.319) (29.3104, 10.3206) (29.3035, 10.3222) (29.2967, 10.3238) (29.2899, 10.3253) (29.2831, 10.3269) (29.2764, 10.3284) (29.2698, 10.3298) (29.2632, 10.3313) (29.2567, 10.3327) (29.2502, 10.3341) (29.2438, 10.3355) (29.2374, 10.3369) (29.2311, 10.3382) (29.2249, 10.3395) (29.2187, 10.3408) (29.2126, 10.3421) (29.2065, 10.3433) (29.2005, 10.3446) (29.1946, 10.3458) (29.1887, 10.347) (29.1829, 10.3481) (29.1771, 10.3493) (29.1714, 10.3504) (29.1658, 10.3515) (29.1602, 10.3525) (29.1547, 10.3536) (29.1493, 10.3546) (29.1439, 10.3556) (29.1386, 10.3566) (29.1334, 10.3576) (29.1282, 10.3585) (29.1231, 10.3594) (29.118, 10.3603) (29.1131, 10.3612) (29.1081, 10.362) (29.1033, 10.3629) (29.0985, 10.3637) (29.0938, 10.3645) (29.0892, 10.3653) (29.0847, 10.366) (29.0802, 10.3668) (29.0758, 10.3675) (29.0714, 10.3682) (29.0672, 10.3688) (29.063, 10.3695) (29.0589, 10.3701) (29.0549, 10.3708) (29.0509, 10.3714) (29.047, 10.3719) (29.0432, 10.3725) (29.0395, 10.373) (29.0359, 10.3736) (29.0323, 10.3741) (29.0289, 10.3746) (29.0255, 10.375) (29.0222, 10.3755) (29.0189, 10.3759) (29.0158, 10.3763) (29.0128, 10.3767) (29.0098, 10.3771) (29.0069, 10.3775) (29.0041, 10.3778) (29.0015, 10.3781) (28.9989, 10.3785) (28.9963, 10.3788) (28.9939, 10.379) (28.9916, 10.3793) (28.9894, 10.3796) (28.9873, 10.3798) (28.9852, 10.38) (28.9833, 10.3802) (28.9815, 10.3804) (28.9798, 10.3806) (28.9781, 10.3808) (28.9766, 10.3809) (28.9752, 10.3811) (28.9739, 10.3812) (28.9727, 10.3813) (28.9716, 10.3814) (28.9706, 10.3815) (28.9698, 10.3816) (28.969, 10.3816) (28.9685, 10.3817) (28.9682, 10.3817) (28.968, 10.3817) (28.9679, 10.3817) knots -1 -1 -1 -1 -1 -1 -0.99583333 -0.99166667 -0.9875 -0.98333333 -0.97916667 -0.975 -0.97083333 -0.96666667 -0.9625 -0.95833333 -0.95416667 -0.95 -0.94583333 -0.94166667 -0.9375 -0.93333333 -0.92916667 -0.925 -0.92083333 -0.91666667 -0.9125 -0.90833333 -0.90416667 -0.9 -0.89583333 -0.89166667 -0.8875 -0.88333333 -0.87916667 -0.875 -0.87083333 -0.86666667 -0.8625 -0.85833333 -0.85416667 -0.85 -0.84583333 -0.84166667 -0.8375 -0.83333333 -0.82916667 -0.825 -0.82083333 -0.81666667 -0.8125 -0.80833333 -0.80416667 -0.8 -0.79583333 -0.79166667 -0.7875 -0.78333333 -0.77916667 -0.775 -0.77083333 -0.76666667 -0.7625 -0.75833333 -0.75416667 -0.75 -0.74583333 -0.74166667 -0.7375 -0.73333333 -0.72916667 -0.725 -0.72083333 -0.71666667 -0.7125 -0.70833333 -0.70416667 -0.7 -0.69583333 -0.69166667 -0.6875 -0.68333333 -0.67916667 -0.675 -0.67083333 -0.66666667 -0.6625 -0.65833333 -0.65416667 -0.65 -0.64583333 -0.64166667 -0.6375 -0.63333333 -0.62916667 -0.625 -0.62083333 -0.61666667 -0.6125 -0.60833333 -0.60416667 -0.6 -0.59583333 -0.59166667 -0.5875 -0.58333333 -0.57916667 -0.575 -0.57083333 -0.56666667 -0.5625 -0.55833333 -0.55416667 -0.55 -0.54583333 -0.54166667 -0.5375 -0.53333333 -0.52916667 -0.525 -0.52083333 -0.51666667 -0.5125 -0.50833333 -0.50416667 -0.5 -0.49583333 -0.49166667 -0.4875 -0.48333333 -0.47916667 -0.475 -0.47083333 -0.46666667 -0.4625 -0.45833333 -0.45416667 -0.45 -0.44583333 -0.44166667 -0.4375 -0.43333333 -0.42916667 -0.425 -0.42083333 -0.41666667 -0.4125 -0.40833333 -0.40416667 -0.4 -0.39583333 -0.39166667 -0.3875 -0.38333333 -0.37916667 -0.375 -0.37083333 -0.36666667 -0.3625 -0.35833333 -0.35416667 -0.35 -0.34583333 -0.34166667 -0.3375 -0.33333333 -0.32916667 -0.325 -0.32083333 -0.31666667 -0.3125 -0.30833333 -0.30416667 -0.3 -0.29583333 -0.29166667 -0.2875 -0.28333333 -0.27916667 -0.275 -0.27083333 -0.26666667 -0.2625 -0.25833333 -0.25416667 -0.25 -0.24583333 -0.24166667 -0.2375 -0.23333333 -0.22916667 -0.225 -0.22083333 -0.21666667 -0.2125 -0.20833333 -0.20416667 -0.2 -0.19583333 -0.19166667 -0.1875 -0.18333333 -0.17916667 -0.175 -0.17083333 -0.16666667 -0.1625 -0.15833333 -0.15416667 -0.15 -0.14583333 -0.14166667 -0.1375 -0.13333333 -0.12916667 -0.125 -0.12083333 -0.11666667 -0.1125 -0.10833333 -0.10416667 -0.1 -0.09583333 -0.09166667 -0.0875 -0.08333333 -0.07916667 -0.075 -0.07083333 -0.06666667 -0.0625 -0.05833333 -0.05416667 -0.05 -0.04583333 -0.04166667 -0.0375 -0.03333333 -0.02916667 -0.025 -0.02083333 -0.01666667 -0.0125 -0.00833333 -0.00416667 0 0 0 0 0 0
  line L135 (28.9679, 10.3817) -> (28.9671, 10.3818)
  line L136 (28.9671, 10.3818) -> (28.6734, 10.4033)
  arc A68 (28.6734, 10.4033) -> (28.7355, 11.5881) centre (0, 12.5) ccw
  line L137 (28.7355, 11.5881) -> (29.0298, 11.5787)
  line L138 (29.0298, 11.5787) -> (29.0307, 11.5787)
  spline S68 degree 5 poles (29.0307, 11.5787) (29.0307, 11.5787) (29.0309, 11.5787) (29.0313, 11.5787) (29.0318, 11.5787) (29.0325, 11.5787) (29.0334, 11.5787) (29.0344, 11.5786) (29.0355, 11.5786) (29.0367, 11.5786) (29.038, 11.5786) (29.0394, 11.5786) (29.0409, 11.5786) (29.0425, 11.5786) (29.0443, 11.5786) (29.0461, 11.5786) (29.0481, 11.5786) (29.0501, 11.5786) (29.0522, 11.5786) (29.0545, 11.5786) (29.0568, 11.5786) (29.0592, 11.5787) (29.0618, 11.5787) (29.0644, 11.5788) (29.0671, 11.5788) (29.0699, 11.5789) (29.0728, 11.5789) (29.0758, 11.579) (29.0788, 11.5791) (29.082, 11.5792) (29.0852, 11.5792) (29.0886, 11.5794) (29.092, 11.5795) (29.0955, 11.5796) (29.0991, 11.5797) (29.1028, 11.5799) (29.1065, 11.58) (29.1103, 11.5802) (29.1143, 11.5803) (29.1183, 11.5805) (29.1223, 11.5807) (29.1265, 11.5809) (29.1307, 11.5811) (29.135, 11.5814) (29.1394, 11.5816) (29.1439, 11.5818) (29.1484, 11.5821) (29.153, 11.5824) (29.1577, 11.5827) (29.1624, 11.583) (29.1673, 11.5833) (29.1722, 11.5836) (29.1771, 11.5839) (29.1822, 11.5843) (29.1873, 11.5847) (29.1925, 11.585) (29.1977, 11.5854) (29.203, 11.5859) (29.2084, 11.5863) (29.2139, 11.5867) (29.2194, 11.5872) (29.225, 11.5876) (29.2306, 11.5881) (29.2363, 11.5886) (29.2421, 11.5891) (29.248, 11.5897) (29.2539, 11.5902) (29.2599, 11.5908) (29.2659, 11.5913) (29.272, 11.5919) (29.2781, 11.5925) (29.2844, 11.5932) (29.2906, 11.5938) (29.297, 11.5945) (29.3034, 11.5951) (29.3099, 11.5958) (29.3164, 11.5965) (29.323, 11.5973) (29.3296, 11.598) (29.3363, 11.5988) (29.343, 11.5995) (29.3498, 11.6003) (29.3567, 11.6011) (29.3636, 11.602) (29.3706, 11.6028) (29.3777, 11.6037) (29.3847, 11.6046) (29.3919, 11.6055) (29.3991, 11.6064) (29.4063, 11.6073) (29.4137, 11.6083) (29.421, 11.6093) (29.4284, 11.6103) (29.4359, 11.6113) (29.4434, 11.6123) (29.451, 11.6134) (29.4586, 11.6144) (29.4663, 11.6155) (29.474, 11.6166) (29.4818, 11.6178) (29.4896, 11.6189) (29.4975, 11.6201) (29.5054, 11.6213) (29.5134, 11.6225) (29.5214, 11.6237) (29.5295, 11.625) (29.5376, 11.6262) (29.5458, 11.6275) (29.554, 11.6288) (29.5623, 11.6302) (29.5706, 11.6315) (29.5789, 11.6329) (29.5873, 11.6343) (29.5958, 11.6357) (29.6043, 11.6371) (29.6128, 11.6386) (29.6214, 11.64) (29.6301, 11.6415) (29.6388, 11.6431) (29.6475, 11.6446) (29.6563, 11.6462) (29.6651, 11.6477) (29.6739, 11.6493) (29.6828, 11.651) (29.6918, 11.6526) (29.7008, 11.6543) (29.7098, 11.656) (29.7189, 11.6577) (29.728, 11.6594) (29.7372, 11.6612) (29.7464, 11.6629) (29.7556, 11.6647) (29.7649, 11.6666) (29.7742, 11.6684) (29.7836, 11.6703) (29.793, 11.6721) (29.8025, 11.6741) (29.812, 11.676) (29.8215, 11.6779) (29.8311, 11.6799) (29.8407, 11.6819) (29.8503, 11.6839) (29.86, 11.686) (29.8697, 11.688) (29.8795, 11.6901) (29.8893, 11.6922) (29.8992, 11.6944) (29.909, 11.6965) (29.919, 11.6987) (29.9289, 11.7009) (29.9389, 11.7031) (29.949, 11.7054) (29.959, 11.7077) (29.9691, 11.71) (29.9793, 11.7123) (29.9895, 11.7146) (29.9997, 11.717) (30.0099, 11.7194) (30.0202, 11.7218) (30.0306, 11.7242) (30.0409, 11.7267) (30.0513, 11.7292) (30.0618, 11.7317) (30.0722, 11.7342) (30.0827, 11.7368) (30.0933, 11.7394) (30.1038, 11.742) (30.1145, 11.7446) (30.1251, 11.7472) (30.1358, 11.7499) (30.1465, 11.7526) (30.1572, 11.7553) (30.168, 11.7581) (30.1788, 11.7609) (30.1897, 11.7636) (30.2005, 11.7665) (30.2114, 11.7693) (30.2224, 11.7722) (30.2334, 11.7751) (30.2444, 11.778) (30.2554, 11.7809) (30.2665, 11.7839) (30.2776, 11.7869) (30.2887, 11.7899) (30.2999, 11.7929) (30.3111, 11.796) (30.3223, 11.7991) (30.3336, 11.8022) (30.3448, 11.8053) (30.3562, 11.8085) (30.3675, 11.8117) (30.3789, 11.8149) (30.3903, 11.8181) (30.4017, 11.8214) (30.4132, 11.8247) (30.4247, 11.828) (30.4362, 11.8313) (30.4478, 11.8347) (30.4594, 11.8381) (30.471, 11.8415) (30.4827, 11.8449) (30.4943, 11.8484) (30.506, 11.8519) (30.5178, 11.8554) (30.5295, 11.8589) (30.5413, 11.8625) (30.5531, 11.8661) (30.565, 11.8697) (30.5769, 11.8733) (30.5888, 11.877) (30.6007, 11.8807) (30.6126, 11.8844) (30.6246, 11.8882) (30.6366, 11.8919) (30.6487, 11.8957) (30.6607, 11.8995) (30.6728, 11.9034) (30.685, 11.9073) (30.6971, 11.9111) (30.7093, 11.9151) (30.7215, 11.919) (30.7337, 11.923) (30.7459, 11.927) (30.7582, 11.931) (30.7705, 11.9351) (30.7828, 11.9391) (30.7952, 11.9432) (30.8076, 11.9474) (30.82, 11.9515) (30.8324, 11.9557) (30.8448, 11.9599) (30.8573, 11.9641) (30.8698, 11.9684) (30.8823, 11.9727) (30.8949, 11.977) (30.9075, 11.9813) (30.9201, 11.9857) (30.9327, 11.9901) (30.9453, 11.9945) (30.958, 11.9989) (30.9707, 12.0034) (30.9809, 12.007) (30.9885, 12.0097) (30.9936, 12.0115) (30.9962, 12.0124) knots 0 0 0 0 0 0 0.00416667 0.00833333 0.0125 0.01666667 0.02083333 0.025 0.02916667 0.03333333 0.0375 0.04166667 0.04583333 0.05 0.05416667 0.05833333 0.0625 0.06666667 0.07083333 0.075 0.07916667 0.08333333 0.0875 0.09166667 0.09583333 0.1 0.10416667 0.10833333 0.1125 0.11666667 0.12083333 0.125 0.12916667 0.13333333 0.1375 0.14166667 0.14583333 0.15 0.15416667 0.15833333 0.1625 0.16666667 0.17083333 0.175 0.17916667 0.18333333 0.1875 0.19166667 0.19583333 0.2 0.20416667 0.20833333 0.2125 0.21666667 0.22083333 0.225 0.22916667 0.23333333 0.2375 0.24166667 0.24583333 0.25 0.25416667 0.25833333 0.2625 0.26666667 0.27083333 0.275 0.27916667 0.28333333 0.2875 0.29166667 0.29583333 0.3 0.30416667 0.30833333 0.3125 0.31666667 0.32083333 0.325 0.32916667 0.33333333 0.3375 0.34166667 0.34583333 0.35 0.35416667 0.35833333 0.3625 0.36666667 0.37083333 0.375 0.37916667 0.38333333 0.3875 0.39166667 0.39583333 0.4 0.40416667 0.40833333 0.4125 0.41666667 0.42083333 0.425 0.42916667 0.43333333 0.4375 0.44166667 0.44583333 0.45 0.45416667 0.45833333 0.4625 0.46666667 0.47083333 0.475 0.47916667 0.48333333 0.4875 0.49166667 0.49583333 0.5 0.50416667 0.50833333 0.5125 0.51666667 0.52083333 0.525 0.52916667 0.53333333 0.5375 0.54166667 0.54583333 0.55 0.55416667 0.55833333 0.5625 0.56666667 0.57083333 0.575 0.57916667 0.58333333 0.5875 0.59166667 0.59583333 0.6 0.60416667 0.60833333 0.6125 0.61666667 0.62083333 0.625 0.62916667 0.63333333 0.6375 0.64166667 0.64583333 0.65 0.65416667 0.65833333 0.6625 0.66666667 0.67083333 0.675 0.67916667 0.68333333 0.6875 0.69166667 0.69583333 0.7 0.70416667 0.70833333 0.7125 0.71666667 0.72083333 0.725 0.72916667 0.73333333 0.7375 0.74166667 0.74583333 0.75 0.75416667 0.75833333 0.7625 0.76666667 0.77083333 0.775 0.77916667 0.78333333 0.7875 0.79166667 0.79583333 0.8 0.80416667 0.80833333 0.8125 0.81666667 0.82083333 0.825 0.82916667 0.83333333 0.8375 0.84166667 0.84583333 0.85 0.85416667 0.85833333 0.8625 0.86666667 0.87083333 0.875 0.87916667 0.88333333 0.8875 0.89166667 0.89583333 0.9 0.90416667 0.90833333 0.9125 0.91666667 0.92083333 0.925 0.92916667 0.93333333 0.9375 0.94166667 0.94583333 0.95 0.95416667 0.95833333 0.9625 0.96666667 0.97083333 0.975 0.97916667 0.98333333 0.9875 0.99166667 0.99583333 1 1 1 1 1 1
  arc A69 (30.9962, 12.0124) -> (30.9962, 12.9876) centre (0, 12.5) ccw
  spline S69 degree 5 poles (30.9962, 12.9876) (30.9936, 12.9885) (30.9885, 12.9903) (30.9809, 12.993) (30.9707, 12.9966) (30.958, 13.0011) (30.9453, 13.0055) (30.9327, 13.0099) (30.9201, 13.0143) (30.9075, 13.0187) (30.8949, 13.023) (30.8823, 13.0273) (30.8698, 13.0316) (30.8573, 13.0359) (30.8448, 13.0401) (30.8324, 13.0443) (30.82, 13.0485) (30.8076, 13.0526) (30.7952, 13.0568) (30.7828, 13.0609) (30.7705, 13.0649) (30.7582, 13.069) (30.7459, 13.073) (30.7337, 13.077) (30.7215, 13.081) (30.7093, 13.0849) (30.6971, 13.0889) (30.685, 13.0927) (30.6728, 13.0966) (30.6607, 13.1005) (30.6487, 13.1043) (30.6366, 13.1081) (30.6246, 13.1118) (30.6126, 13.1156) (30.6007, 13.1193) (30.5888, 13.123) (30.5769, 13.1267) (30.565, 13.1303) (30.5531, 13.1339) (30.5413, 13.1375) (30.5295, 13.1411) (30.5178, 13.1446) (30.506, 13.1481) (30.4943, 13.1516) (30.4827, 13.1551) (30.471, 13.1585) (30.4594, 13.1619) (30.4478, 13.1653) (30.4362, 13.1687) (30.4247, 13.172) (30.4132, 13.1753) (30.4017, 13.1786) (30.3903, 13.1819) (30.3789, 13.1851) (30.3675, 13.1883) (30.3562, 13.1915) (30.3448, 13.1947) (30.3336, 13.1978) (30.3223, 13.2009) (30.3111, 13.204) (30.2999, 13.2071) (30.2887, 13.2101) (30.2776, 13.2131) (30.2665, 13.2161) (30.2554, 13.2191) (30.2444, 13.222) (30.2334, 13.2249) (30.2224, 13.2278) (30.2114, 13.2307) (30.2005, 13.2335) (30.1897, 13.2364) (30.1788, 13.2391) (30.168, 13.2419) (30.1572, 13.2447) (30.1465, 13.2474) (30.1358, 13.2501) (30.1251, 13.2528) (30.1145, 13.2554) (30.1038, 13.258) (30.0933, 13.2606) (30.0827, 13.2632) (30.0722, 13.2658) (30.0618, 13.2683) (30.0513, 13.2708) (30.0409, 13.2733) (30.0306, 13.2758) (30.0202, 13.2782) (30.0099, 13.2806) (29.9997, 13.283) (29.9895, 13.2854) (29.9793, 13.2877) (29.9691, 13.29) (29.959, 13.2923) (29.949, 13.2946) (29.9389, 13.2969) (29.9289, 13.2991) (29.919, 13.3013) (29.909, 13.3035) (29.8992, 13.3056) (29.8893, 13.3078) (29.8795, 13.3099) (29.8697, 13.312) (29.86, 13.314) (29.8503, 13.3161) (29.8407, 13.3181) (29.8311, 13.3201) (29.8215, 13.3221) (29.812, 13.324) (29.8025, 13.3259) (29.793, 13.3279) (29.7836, 13.3297) (29.7742, 13.3316) (29.7649, 13.3334) (29.7556, 13.3353) (29.7464, 13.3371) (29.7372, 13.3388) (29.728, 13.3406) (29.7189, 13.3423) (29.7098, 13.344) (29.7008, 13.3457) (29.6918, 13.3474) (29.6828, 13.349) (29.6739, 13.3507) (29.6651, 13.3523) (29.6563, 13.3538) (29.6475, 13.3554) (29.6388, 13.3569) (29.6301, 13.3585) (29.6214, 13.36) (29.6128, 13.3614) (29.6043, 13.3629) (29.5958, 13.3643) (29.5873, 13.3657) (29.5789, 13.3671) (29.5706, 13.3685) (29.5623, 13.3698) (29.554, 13.3712) (29.5458, 13.3725) (29.5376, 13.3738) (29.5295, 13.375) (29.5214, 13.3763) (29.5134, 13.3775) (29.5054, 13.3787) (29.4975, 13.3799) (29.4896, 13.3811) (29.4818, 13.3822) (29.474, 13.3834) (29.4663, 13.3845) (29.4586, 13.3856) (29.451, 13.3866) (29.4434, 13.3877) (29.4359, 13.3887) (29.4284, 13.3897) (29.421, 13.3907) (29.4137, 13.3917) (29.4063, 13.3927) (29.3991, 13.3936) (29.3919, 13.3945) (29.3847, 13.3954) (29.3777, 13.3963) (29.3706, 13.3972) (29.3636, 13.398) (29.3567, 13.3989) (29.3498, 13.3997) (29.343, 13.4005) (29.3363, 13.4012) (29.3296, 13.402) (29.323, 13.4027) (29.3164, 13.4035) (29.3099, 13.4042) (29.3034, 13.4049) (29.297, 13.4055) (29.2906, 13.4062) (29.2844, 13.4068) (29.2781, 13.4075) (29.272, 13.4081) (29.2659, 13.4087) (29.2599, 13.4092) (29.2539, 13.4098) (29.248, 13.4103) (29.2421, 13.4109) (29.2363, 13.4114) (29.2306, 13.4119) (29.225, 13.4124) (29.2194, 13.4128) (29.2139, 13.4133) (29.2084, 13.4137) (29.203, 13.4141) (29.1977, 13.4146) (29.1925, 13.415) (29.1873, 13.4153) (29.1822, 13.4157) (29.1771, 13.4161) (29.1722, 13.4164) (29.1673, 13.4167) (29.1624, 13.417) (29.1577, 13.4173) (29.153, 13.4176) (29.1484, 13.4179) (29.1439, 13.4182) (29.1394, 13.4184) (29.135, 13.4186) (29.1307, 13.4189) (29.1265, 13.4191) (29.1223, 13.4193) (29.1183, 13.4195) (29.1143, 13.4197) (29.1103, 13.4198) (29.1065, 13.42) (29.1028, 13.4201) (29.0991, 13.4203) (29.0955, 13.4204) (29.092, 13.4205) (29.0886, 13.4206) (29.0852, 13.4208) (29.082, 13.4208) (29.0788, 13.4209) (29.0758, 13.421) (29.0728, 13.4211) (29.0699, 13.4211) (29.0671, 13.4212) (29.0644, 13.4212) (29.0618, 13.4213) (29.0592, 13.4213) (29.0568, 13.4214) (29.0545, 13.4214) (29.0522, 13.4214) (29.0501, 13.4214) (29.0481, 13.4214) (29.0461, 13.4214) (29.0443, 13.4214) (29.0425, 13.4214) (29.0409, 13.4214) (29.0394, 13.4214) (29.038, 13.4214) (29.0367, 13.4214) (29.0355, 13.4214) (29.0344, 13.4214) (29.0334, 13.4213) (29.0325, 13.4213) (29.0318, 13.4213) (29.0313, 13.4213) (29.0309, 13.4213) (29.0307, 13.4213) (29.0307, 13.4213) knots -1 -1 -1 -1 -1 -1 -0.99583333 -0.99166667 -0.9875 -0.98333333 -0.97916667 -0.975 -0.97083333 -0.96666667 -0.9625 -0.95833333 -0.95416667 -0.95 -0.94583333 -0.94166667 -0.9375 -0.93333333 -0.92916667 -0.925 -0.92083333 -0.91666667 -0.9125 -0.90833333 -0.90416667 -0.9 -0.89583333 -0.89166667 -0.8875 -0.88333333 -0.87916667 -0.875 -0.87083333 -0.86666667 -0.8625 -0.85833333 -0.85416667 -0.85 -0.84583333 -0.84166667 -0.8375 -0.83333333 -0.82916667 -0.825 -0.82083333 -0.81666667 -0.8125 -0.80833333 -0.80416667 -0.8 -0.79583333 -0.79166667 -0.7875 -0.78333333 -0.77916667 -0.775 -0.77083333 -0.76666667 -0.7625 -0.75833333 -0.75416667 -0.75 -0.74583333 -0.74166667 -0.7375 -0.73333333 -0.72916667 -0.725 -0.72083333 -0.71666667 -0.7125 -0.70833333 -0.70416667 -0.7 -0.69583333 -0.69166667 -0.6875 -0.68333333 -0.67916667 -0.675 -0.67083333 -0.66666667 -0.6625 -0.65833333 -0.65416667 -0.65 -0.64583333 -0.64166667 -0.6375 -0.63333333 -0.62916667 -0.625 -0.62083333 -0.61666667 -0.6125 -0.60833333 -0.60416667 -0.6 -0.59583333 -0.59166667 -0.5875 -0.58333333 -0.57916667 -0.575 -0.57083333 -0.56666667 -0.5625 -0.55833333 -0.55416667 -0.55 -0.54583333 -0.54166667 -0.5375 -0.53333333 -0.52916667 -0.525 -0.52083333 -0.51666667 -0.5125 -0.50833333 -0.50416667 -0.5 -0.49583333 -0.49166667 -0.4875 -0.48333333 -0.47916667 -0.475 -0.47083333 -0.46666667 -0.4625 -0.45833333 -0.45416667 -0.45 -0.44583333 -0.44166667 -0.4375 -0.43333333 -0.42916667 -0.425 -0.42083333 -0.41666667 -0.4125 -0.40833333 -0.40416667 -0.4 -0.39583333 -0.39166667 -0.3875 -0.38333333 -0.37916667 -0.375 -0.37083333 -0.36666667 -0.3625 -0.35833333 -0.35416667 -0.35 -0.34583333 -0.34166667 -0.3375 -0.33333333 -0.32916667 -0.325 -0.32083333 -0.31666667 -0.3125 -0.30833333 -0.30416667 -0.3 -0.29583333 -0.29166667 -0.2875 -0.28333333 -0.27916667 -0.275 -0.27083333 -0.26666667 -0.2625 -0.25833333 -0.25416667 -0.25 -0.24583333 -0.24166667 -0.2375 -0.23333333 -0.22916667 -0.225 -0.22083333 -0.21666667 -0.2125 -0.20833333 -0.20416667 -0.2 -0.19583333 -0.19166667 -0.1875 -0.18333333 -0.17916667 -0.175 -0.17083333 -0.16666667 -0.1625 -0.15833333 -0.15416667 -0.15 -0.14583333 -0.14166667 -0.1375 -0.13333333 -0.12916667 -0.125 -0.12083333 -0.11666667 -0.1125 -0.10833333 -0.10416667 -0.1 -0.09583333 -0.09166667 -0.0875 -0.08333333 -0.07916667 -0.075 -0.07083333 -0.06666667 -0.0625 -0.05833333 -0.05416667 -0.05 -0.04583333 -0.04166667 -0.0375 -0.03333333 -0.02916667 -0.025 -0.02083333 -0.01666667 -0.0125 -0.00833333 -0.00416667 0 0 0 0 0 0
  line L139 (29.0307, 13.4213) -> (29.0298, 13.4213)
  line L140 (29.0298, 13.4213) -> (28.7355, 13.4119)
  arc A70 (28.7355, 13.4119) -> (28.6734, 14.5967) centre (0, 12.5) ccw
  line L141 (28.6734, 14.5967) -> (28.9671, 14.6182)
  line L142 (28.9671, 14.6182) -> (28.9679, 14.6183)